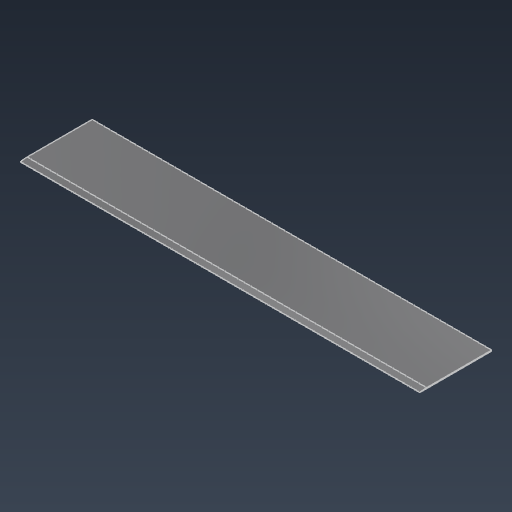
# Autodesk Inventor part: plog
Saved by Autodesk Inventor 2023 (Build 270158000, 158)
## iProperties
Created: 2025-04-27
Part Number: plog
Material: Stainless Steel
Document SubType Name: Modeling
Designer: szymo
Density: 8 g/cm^3
Appearance: Silicon Nitride - Polished
Mass: 2.0415 g
Surface Area: 27.2385 cm^2
Volume: 0.255187 cm^3
Author: szymo
Autodesk Inventor part; units mm, degrees
ref_plane "YZ Plane" through (0, 0, 0) normal (1, 0, 0) x (0, 1, 0)
ref_plane "XZ Plane" through (0, 0, 0) normal (0, 1, 0) x (-1, 0, 0)
ref_plane "XY Plane" through (0, 0, 0) normal (0, 0, 1) x (1, 0, 0)
sketch "Sketch1" plane through (0, 0, 0) normal (0, 1, 0) x (-1, 0, 0)
  line L0 (50, 9) -> (-50, 9)
  line L1 (-50, 9) -> (-50, -9)
  line L2 (-50, -9) -> (50, -9)
  line L3 (50, -9) -> (50, 9)
  line L4 (50, 9) -> (-50, -9) construction
  line L5 (-50, 9) -> (50, -9) construction
  point P0 (0, 0)
  point P1 (0, 0)
  dimension "d0" = 18
  dimension "d1" = 100
  constraints: 12 end point, 2 midpoint, 2 parallel, 1 coincident, 1 horizontal, 1 perpendicular
  measures "d0" distance of L2.end L0.start
  measures "d1" distance of L1.end L2.end
extrude "Extrusion1" add sketch "Sketch1" along normal blind 0.2
chamfer "Chamfer1" distance 0.15 angle 85 1 edges at (0, 0.2, 9) measured on face at (0, 0.1, 9)
ref_plane "Work Plane1" through (-17.675, -5.5815, -6.7023) normal (0, 0.9191353, 0.3939419) x (1, 0, 0)
body "Solid1"
